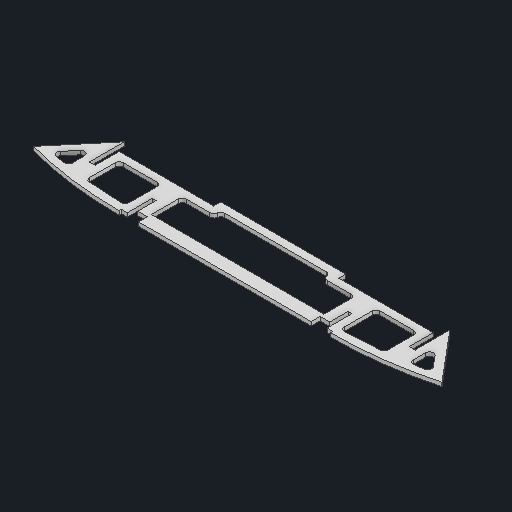
# Autodesk Inventor part: tail_1
Saved by Autodesk Inventor 2023 (Build 270158030, 158C)
## iProperties
Created: 2022-03-21
Part Number: tail_1
Material: Generic
Document SubType Name: Modeling
Designer: kardo
Density: 1 g/cm^3
Appearance: Default
Mass: 2.78715 g
Surface Area: 39.0166 cm^2
Volume: 2.78715 cm^3
Author: kardo
Autodesk Inventor part; units mm, degrees
ref_plane "YZ Plane" through (0, 0, 0) normal (1, 0, 0) x (0, 1, 0)
ref_plane "XZ Plane" through (0, 0, 0) normal (0, 1, 0) x (-1, 0, 0)
ref_plane "XY Plane" through (0, 0, 0) normal (0, 0, 1) x (1, 0, 0)
derived "parameters_frame.ipt"
derived "stencil_frame.ipt"
sketch "sk_joint_locations" plane through (81.12, 0, 0) normal (1, 0, 0) x (0, 1, 0)
  line L0 (0, 0) -> (122.4, 8.559) construction
  line L1 (36.465, 28.832) -> (112.2, 28.832) construction
  arc A0 (36.465, 28.832) -> (11.22, 28.376) centre (36.465, -670.197) ccw construction
  line L2 (-241.5001, 19.2432) -> (11.22, 28.376) construction
  line L3 (-345, 16.32) -> (-262.2001, 18.586) construction
  arc A1 (-262.2001, 18.586) -> (-241.5001, 19.2432) centre (-326.8578, 2381.2399) ccw construction
  line L4 (-95.1358, 3119.4657) -> (254.2444, -1876.9042) construction
  line L5 (-230.0001, 3089.1136) -> (-230.0001, -1866.0023) construction
  line L6 (-114.9999, 3089.1136) -> (-114.9999, -1866.0023) construction
  line L7 (-345, 3089.1136) -> (-345, -1866.0023) construction
  line L8 (0, 3089.1136) -> (0, -1866.0023) construction
  line L9 (516.4305, 45.5774) -> (-594.5903, 6.7797) construction
  line L10 (-657.7604, -27.3784) -> (621.8174, 62.0984) construction
  line L11 (193.4506, 30.2962) -> (193.1714, 38.2913) construction
  line L12 (201.1621, 36.7028) -> (201.7215, 28.7028) construction
  line L13 (0, 14.96) -> (121.9304, 15.2746) construction
  line L14 (-230.0001, 45.8702) -> (-230.0001, 19.6588) construction
  line L15 (-345, 37.4554) -> (-345, 16.32) construction
  line L16 (-114.9999, 51.0173) -> (-114.9999, 23.8147) construction
  line L17 (0, 52.89) -> (0, 27.9705) construction
  line L18 (119.462, 50.575) -> (119.9556, 43.5149) construction
  line L19 (120.4493, 36.4549) -> (119.9556, 43.5149) construction
  line L20 (120.4493, 36.4549) -> (120.943, 29.3948) construction
  line L21 (120.943, 29.3948) -> (121.4367, 22.3347) construction
  line L22 (121.4367, 22.3347) -> (121.9304, 15.2746) construction
  line L23 (0, 14.96) -> (0, 0) construction
  spline S0 degree 4 poles (-345, 37.4554) (-258.8682, 45.1562) (-172.5926, 49.7838) (-86.3161, 52.89) (0, 52.89) knots 0 0 0 0 0 1 1 1 1 1
  spline S1 degree 3 poles (0, 52.89) (92.8353, 52.89) (195.0311, 49.5089) (255, 36.448) knots 0 0 0 0 1 1 1 1
  spline S2 degree 2 poles (122.4, 8.559) (190.3044, 13.3074) (255, 36.448) knots 0 0 0 1 1 1
  line L24 (112.2, 37.536) -> (112.2, 28.832) construction
  line L25 (112.2, 35.548) -> (112.2, 30.82) construction
  point P0 (-95.1358, 3119.4657)
  point P1 (254.2444, -1876.9042)
  point P2 (193.311, 34.2938)
  point P3 (201.4418, 32.7028)
  point P4 (134.9575, 11.3411)
  point P5 (-345, 26.8877)
  point P6 (-230.0001, 32.7645)
  point P7 (-114.9999, 37.416)
  point P8 (0, 40.4303)
  point P9 (112.2, 33.184)
sketch "sk_cowl_joint_locations" plane through (54.6, 0, 0) normal (1, 0, 0) x (0, 1, 0)
  line L0 (-345, 16.32) -> (-262.2001, 18.586) construction
  arc A0 (-262.2001, 18.586) -> (-241.5001, 19.2432) centre (-326.8578, 2381.2399) ccw construction
  line L1 (-241.5001, 19.2432) -> (11.22, 28.376) construction
  arc A1 (36.465, 28.832) -> (11.22, 28.376) centre (36.465, -670.197) ccw construction
  line L2 (36.465, 28.832) -> (112.2, 28.832) construction
  line L3 (94.8, 30.032) -> (36.465, 30.032) construction
  arc A2 (36.465, 30.032) -> (11.1767, 29.5752) centre (36.465, -670.197) ccw construction
  line L4 (11.1767, 29.5752) -> (-241.5434, 20.4424) construction
  arc A3 (-262.2329, 19.7855) -> (-241.5434, 20.4424) centre (-326.8578, 2381.2399) ccw construction
  line L5 (-262.2329, 19.7855) -> (-345, 17.5204) construction
  line L6 (-230.0001, 3089.1136) -> (-230.0001, -1866.0023) construction
  line L7 (-114.9999, 3089.1136) -> (-114.9999, -1866.0023) construction
  line L8 (-345, 3089.1136) -> (-345, -1866.0023) construction
  line L9 (0, 3089.1136) -> (0, -1866.0023) construction
  line L10 (-230.0001, 45.0685) -> (-230.0001, 20.8596) construction
  line L11 (-114.9999, 49.9659) -> (-114.9999, 25.0155) construction
  line L12 (-345, 17.5204) -> (-345, 17.5204)
  line L13 (-345, 17.5204) -> (-345, 36.9221) construction
  line L14 (-869.78, 3004.1953) -> (348.339, -1881.413) construction
  line L15 (-344.7623, 36.9221) -> (-345, 39.712) construction
  line L16 (0, 51.6) -> (0, 29.1713) construction
  spline S0 degree 2 poles (-345, 39.712) (-172.656, 54.3934) (0, 54.4) knots 0 0 0 1 1 1
  spline S1 degree 3 poles (0, 54.4) (37.026, 54.4) (80.784, 47.9917) (112.2, 37.536) knots 1 1 1 1 2 2 2 2
  spline S2 degree 3 poles (111.3158, 34.8793) (106.1488, 36.5989) (96.4909, 39.4217) (84.5445, 42.2265) (75.2974, 44.1359) (69.0059, 45.3094) (61.0256, 46.6466) (54.5653, 47.6105) (46.4371, 48.6777) (39.9092, 49.4192) (31.7597, 50.2005) (25.2653, 50.7072) (17.2211, 51.1873) (9.2717, 51.5118) (3.0586, 51.6) (0, 51.6) knots 1 1 1 1 1.166667 1.291667 1.333333 1.416667 1.458333 1.541667 1.583333 1.666667 1.708333 1.791667 1.833333 1.916667 2 2 2 2
  spline S3 degree 3 poles (0, 51.6) (-19.1708, 51.5993) (-52.7146, 51.3604) (-91.0402, 50.6121) (-119.7801, 49.8472) (-138.9379, 49.2354) (-162.8824, 48.3434) (-182.0358, 47.528) (-205.975, 46.3814) (-225.1241, 45.3623) (-249.0578, 43.9611) (-268.2026, 42.7383) (-292.131, 41.0825) (-316.0566, 39.2994) (-335.1942, 37.7372) (-344.7623, 36.9221) knots 0 0 0 0 0.166667 0.291667 0.333333 0.416667 0.458333 0.541666 0.583333 0.666666 0.708333 0.791666 0.833333 0.916666 1 1 1 1
  line L17 (-136.2088, 45.4676) -> (-130.9657, 24.4385) construction
  line L18 (-128.3953, 30.6635) -> (-132.2764, 29.6958) construction
  line L19 (-131.0168, 41.178) -> (-134.898, 40.2103) construction
  line L20 (-136.2088, 45.4676) -> (-132.3276, 46.4353) construction
  line L21 (-130.9657, 24.4385) -> (-127.0845, 25.4062) construction
  line L22 (-132.3276, 46.4353) -> (-132.5171, 52.2322) construction
  point P0 (0, 0)
  point P1 (-345, 27.2213)
  point P2 (-230.0001, 32.964)
  point P3 (-114.9999, 37.4907)
  point P4 (0, 40.3857)
  point P5 (-869.78, 3004.1953)
  point P6 (348.339, -1881.413)
  point P7 (-85.2629, 50.788)
  point P8 (0, 40.3857)
sketch "sk_tail_1_base" plane through (0, -114.9999, 0) normal (0, 1, 0) x (-1, 0, 0)
  spline S0 degree 2 poles (-156, 25.0328) (-108.0933, 52.767) (-54.6, 52.767) knots 0 0 0 1 1 1 construction
  line L0 (-54.6, 52.767) -> (0, 52.767) construction
  line L1 (0, -1866.0023) -> (0, 3089.1136) construction
  line L2 (891.2291, -1144.8379) -> (-1640.6009, 1872.4796) construction
  line L3 (-105.5205, 44.909) -> (-84.12, 19.4048)
  line L4 (-84.12, 19.4048) -> (-84.12, 37.416)
  line L5 (-84.12, 37.416) -> (-81.12, 37.416)
  line L6 (-81.12, 37.416) -> (-81.12, 25.0147)
  line L7 (-81.12, 25.0147) -> (-32.32, 25.0147)
  line L8 (-32.32, 25.0147) -> (-32.32, 21.4065)
  line L9 (-32.32, 21.4065) -> (0, 21.4065)
  line L10 (0, 21.4065) -> (0, 51.567)
  line L11 (-54.6, 51.567) -> (0, 51.567)
  spline S1 degree 5 poles (-155.3988, 23.9943) (-146.1642, 29.3403) (-136.6166, 34.1448) (-126.7717, 38.3404) (-106.7544, 45.3182) (-85.9792, 49.5247) (-75.5572, 50.8983) (-65.0787, 51.5669) (-54.6, 51.567) knots 0 0 0 0 0 0 0.504531 0.504531 0.504531 1 1 1 1 1 1
  point P0 (0, 0)
  point P1 (-34.32, 23.8147)
  point P2 (-34.32, 20.2065)
  dimension "d8" = 1.2
  dimension "d3" = 1.2
  dimension "d4" = 1.2
  dimension "d5" = 2
  dimension "d6" = 3
  dimension "d7" = 1.2
  constraints: 18 end point, 5 parallel, 3 perpendicular, 2 point on line, 4 other
  measures "d3" distance from line of point (-34.32, 20.206) L9
  measures "d4" distance from line of L7 point (-34.32, 23.815)
  measures "d5" distance from line of point (-34.32, 23.815) L8
  measures "d6" distance of L4.end L5.end
  measures "d7" distance between parallel lines of L2 L3
extrude "thicken" add sketch "sk_tail_1_base" along normal blind 2
sketch "sk_cut_stringer_cowl" plane through (0, -114.9999, 0) normal (0, 1, 0) x (-1, 0, 0)
  line L0 (-54.6, -1866.0023) -> (-54.6, 3089.1136) construction
  line L1 (-54.6, 52.767) -> (0, 52.767) projected
  line L2 (-49.6, 52.767) -> (-49.6, 37.4907)
  line L3 (-49.6, 37.4907) -> (-51.6, 37.4907)
  line L4 (-51.6, 37.4907) -> (-51.6, 52.767)
  point P0 (0, 0)
  point P1 (-54.6, 37.4907)
  dimension "d11" = 2
  dimension "d12" = 5
  constraints: 6 end point, 3 point on line, 2 parallel
  measures "d11" distance between parallel lines of L4 L2
  measures "d12" distance between parallel lines of L0 L2
extrude "cut_joint" cut sketch "sk_cut_stringer_cowl" along normal through all both and the other way through all
sketch "sk_cut_cowl_liner" plane through (0, -114.9999, 0) normal (0, 1, 0) x (-1, 0, 0)
  line L0 (-54.6, 52.767) -> (0, 52.767) projected
  line L1 (-54.6, -1866.0023) -> (-54.6, 3089.1136) projected
  line L2 (-44.6, 52.767) -> (-44.6, 46.967)
  line L3 (-44.6, 46.967) -> (-49.6, 46.967)
  line L4 (-49.6, 46.967) -> (-49.6, 50.367)
  line L5 (-49.6, 50.367) -> (-54.6, 50.367)
  point P0 (0, 0)
  dimension "d15" = 5
  dimension "d16" = 5
  dimension "d17" = 2.4
  dimension "d38" = 5.8
  constraints: 8 end point, 4 parallel, 2 point on line
  measures "d15" distance between parallel lines of L4 L2
  measures "d16" distance of L4.end L5.end
  measures "d17" distance between parallel lines of L0 L5
  measures "d38" distance of L2.start L2.end
extrude "cut_liner" cut sketch "sk_cut_cowl_liner" along normal through all both and the other way through all
sketch "sk_cut_weight" plane through (0, -114.9999, 0) normal (0, 1, 0) x (-1, 0, 0)
  line L0 (-32.32, 21.4065) -> (0, 21.4065) construction
  line L1 (-32.32, 25.0147) -> (-32.32, 21.4065) construction
  line L2 (-81.12, 25.0147) -> (-32.32, 25.0147) construction
  line L3 (-81.12, 37.416) -> (-81.12, 25.0147) construction
  line L4 (-49.6, 46.967) -> (-49.6, 50.367) construction
  line L5 (-44.6, 46.967) -> (-49.6, 46.967) construction
  line L6 (-44.6, 52.767) -> (-44.6, 46.967) construction
  spline S0 degree 3 poles (-155.3988, 23.9943) (-152.7513, 25.527) (-147.4311, 28.4643) (-140.7179, 31.8161) (-133.9574, 34.928) (-128.5111, 37.2257) (-121.6557, 39.8583) (-116.1333, 41.7727) (-109.1827, 43.9263) (-103.5839, 45.4576) (-96.5374, 47.1325) (-90.8618, 48.2809) (-82.2903, 49.7165) (-70.7585, 51.1202) (-60.5091, 51.567) (-54.6, 51.567) knots 0 0 0 0 0.083333 0.166667 0.208333 0.291667 0.333333 0.416667 0.458333 0.541667 0.583333 0.666667 0.708333 0.833333 1 1 1 1 construction
  line L7 (0, -1866.0023) -> (0, 3089.1136) projected
  line L8 (0, 25.4065) -> (-28.32, 25.4065)
  line L9 (-28.32, 25.4065) -> (-28.32, 29.0147)
  line L10 (-28.32, 29.0147) -> (-44.6, 29.0147)
  line L11 (-77.12, 29.0147) -> (-77.12, 46.3027)
  line L12 (-77.12, 46.3027) -> (-55.6, 47.567)
  line L13 (-55.6, 47.567) -> (-55.6, 29.0147)
  line L14 (-55.6, 29.0147) -> (-77.12, 29.0147)
  line L15 (-44.6, 44.967) -> (-44.6, 29.0147)
  line L16 (-44.6, 44.967) -> (0, 44.967)
  line L17 (-77.12, 46.3027) -> (-77.12, 50.3027) construction
  line L18 (-49.6, 46.967) -> (-49.6, 25.0147) construction
  line L19 (-49.6, 46.967) -> (-51.6, 46.967) construction
  line L20 (-51.6, 46.967) -> (-51.6, 25.0147) construction
  line L21 (-105.5205, 44.909) -> (-84.12, 19.4048) construction
  line L22 (-84.12, 19.4048) -> (-84.12, 37.416) construction
  line L23 (-88.12, 30.3947) -> (-88.12, 44.7341)
  line L24 (-88.12, 44.7341) -> (-98.6522, 42.9465)
  line L25 (-98.6522, 42.9465) -> (-88.12, 30.3947)
  line L26 (-88.12, 44.7341) -> (-88.12, 48.7341) construction
  line L27 (-98.6522, 42.9465) -> (-101.2234, 46.0107) construction
  point P0 (0, 0)
  dimension "d21" = 4
  dimension "d22" = 2
  dimension "d23" = 4
  dimension "d24" = 4
  dimension "d25" = 4
  dimension "d27" = 2
  dimension "d28" = 4
  dimension "d29" = 4
  dimension "d30" = 4
  dimension "d31" = 4
  dimension "d35" = 4
  dimension "d36" = 4
  dimension "d37" = 4
  constraints: 36 end point, 12 parallel, 5 collinear, 4 point on line, 1 equal length, 1 perpendicular, 3 other
  measures "d21" distance of L11.end L17.end
  measures "d22" distance between parallel lines of L20 L18
  measures "d23" distance between parallel lines of L0 L8
  measures "d24" distance between parallel lines of L1 L9
  measures "d25" distance between parallel lines of L10 L2
  measures "d27" distance between parallel lines of L16 L5
  measures "d28" distance between parallel lines of L20 L13
  measures "d29" distance between parallel lines of L2 L14
  measures "d30" distance between parallel lines of L11 L3
  measures "d31" vertical distance of point (-54.6, 51.567) L12.end
  measures "d35" distance between parallel lines of L21 L25
  measures "d36" distance between parallel lines of L23 L22
  measures "d37" distance of L23.end L26.end
extrude "cut_weight" cut sketch "sk_cut_weight" along normal through all both and the other way through all
fillet "round_corners" radius 2 10 edges at (28.32, -113.9999, 25.4065) (28.32, -113.9999, 29.0147) (77.12, -113.9999, 29.0147) (55.6, -113.9999, 29.0147) (44.6, -113.9999, 29.0147) (77.12, -113.9999, 46.3027) (55.6, -113.9999, 47.567) (98.6522, -113.9999, 42.9465) (88.12, -113.9999, 30.3947) (88.12, -113.9999, 44.7341)
mirror "mirror" about plane through (0, 0, 0) normal (1, 0, 0)
equation "\"d8\" = shell_thickness"
equation "\"d3\" = shell_thickness"
equation "\"d4\" = shell_thickness"
equation "\"d5\" = bulkhead_thickness"
equation "\"d6\" = stringer_thickness"
equation "\"d7\" = shell_thickness"
equation "\"d9\" = bulkhead_thickness"
equation "\"d11\" = bulkhead_thickness"
equation "\"d12\" = cowl_liner_width"
equation "\"d15\" = cowl_sealing_width"
equation "\"d16\" = cowl_liner_width"
equation "\"d17\" = shell_thickness + cowl_liner_thickness"
equation "\"d38\" = cowl_sealing_thickness + cowl_shell_thickness + cowl_liner_thickness"
equation "\"d21\" = bulkhead_inset"
equation "\"d22\" = bulkhead_thickness"
equation "\"d23\" = bulkhead_inset"
equation "\"d24\" = bulkhead_inset"
equation "\"d25\" = bulkhead_inset"
equation "\"d28\" = bulkhead_inset"
equation "\"d29\" = bulkhead_inset"
equation "\"d30\" = bulkhead_inset"
equation "\"d31\" = bulkhead_inset"
equation "\"d35\" = bulkhead_inset"
equation "\"d36\" = bulkhead_inset"
equation "\"d37\" = bulkhead_inset"
equation "\"d34\" = 0.5 * bulkhead_inset"
equation "\"shell_thickness\" = 1.2"
equation "\"stringer_thickness\" = 3"
equation "\"bulkhead_thickness\" = 2"
equation "\"cowl_liner_width\" = 5"
equation "\"cowl_sealing_width\" = 5"
equation "\"cowl_liner_thickness\" = 1.2"
equation "\"cowl_sealing_thickness\" = 3"
equation "\"cowl_shell_thickness\" = 1.6"
equation "\"bulkhead_inset\" = 4"
body "Solid1"
